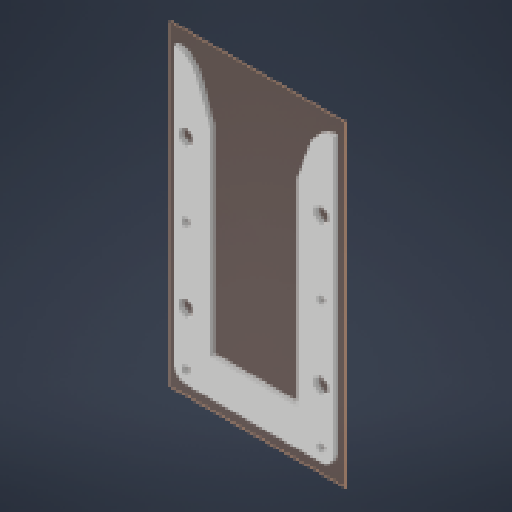
# Autodesk Inventor part: battery holder flap
Saved by Autodesk Inventor 2023 (Build 270158000, 158)
## iProperties
Created: 2022-06-04
Part Number: battery holder flap
Material: Generic
Document SubType Name: Modeling
Designer: vibhu
Density: 1 g/cm^3
Appearance: Default
Author: vibhu
Autodesk Inventor part; units mm, degrees
ref_plane "YZ Plane" through (0, 0, 0) normal (1, 0, 0) x (0, 1, 0)
ref_plane "XZ Plane" through (0, 0, 0) normal (0, 1, 0) x (-1, 0, 0)
ref_plane "XY Plane" through (0, 0, 0) normal (0, 0, 1) x (1, 0, 0)
ref_plane "Work Plane1" through (0, 0, 0) normal (0, 0, 1) x (1, 0, 0)
sketch "Sketch1" plane through (0, 0, 0) normal (0, 0, 1) x (1, 0, 0)
  line L0 (30.3146, 30.125) -> (30.3146, 26.875) projected
  line L1 (30.3146, 26.875) -> (27.5, 25.25) projected
  line L2 (27.5, 25.25) -> (24.6854, 26.875) projected
  line L3 (24.6854, 26.875) -> (24.6854, 30.125) projected
  line L4 (24.6854, 30.125) -> (27.5, 31.75) projected
  line L5 (27.5, 31.75) -> (30.3146, 30.125) projected
  line L6 (30.3146, -33.125) -> (27.5, -34.75) projected
  line L7 (27.5, -34.75) -> (24.6854, -33.125) projected
  line L8 (24.6854, -33.125) -> (24.6854, -29.875) projected
  line L9 (24.6854, -29.875) -> (27.5, -28.25) projected
  line L10 (27.5, -28.25) -> (30.3146, -29.875) projected
  line L11 (30.3146, -29.875) -> (30.3146, -33.125) projected
  line L12 (-24.6854, 26.875) -> (-27.5, 25.25) projected
  line L13 (-27.5, 25.25) -> (-30.3146, 26.875) projected
  line L14 (-30.3146, 26.875) -> (-30.3146, 30.125) projected
  line L15 (-30.3146, 30.125) -> (-27.5, 31.75) projected
  line L16 (-27.5, 31.75) -> (-24.6854, 30.125) projected
  line L17 (-24.6854, 30.125) -> (-24.6854, 26.875) projected
  line L18 (-24.6854, -33.125) -> (-27.5, -34.75) projected
  line L19 (-27.5, -34.75) -> (-30.3146, -33.125) projected
  line L20 (-30.3146, -33.125) -> (-30.3146, -29.875) projected
  line L21 (-30.3146, -29.875) -> (-27.5, -28.25) projected
  line L22 (-27.5, -28.25) -> (-24.6854, -29.875) projected
  line L23 (-24.6854, -29.875) -> (-24.6854, -33.125) projected
  line L24 (-32.5, -53.5) -> (-32.5, 58.5) projected
  arc A0 (-32.5, -53.5) -> (-27.5, -58.5) centre (-27.5, -53.5) ccw projected
  line L25 (27.5, -58.5) -> (-27.5, -58.5) projected
  arc A1 (27.5, -58.5) -> (32.5, -53.5) centre (27.5, -53.5) ccw projected
  line L26 (32.5, 58.5) -> (32.5, -53.5) projected
  arc A2 (32.5, 58.5) -> (22.5, 48.5) centre (32.5, 48.5) ccw projected
  line L27 (22.5, -48.5) -> (22.5, 48.5) projected
  line L28 (-22.5, -48.5) -> (22.5, -48.5) projected
  line L29 (-22.5, 48.5) -> (-22.5, -48.5) projected
  arc A3 (-22.5, 48.5) -> (-32.5, 58.5) centre (-32.5, 48.5) ccw projected
  circle A4 centre (27.5, -1.5) radius 1.75 projected
  circle A5 centre (-27.5, -1.5) radius 1.75 projected
  circle A6 centre (-27.5, -53.5) radius 1.75 projected
  circle A7 centre (27.5, -53.5) radius 1.75 projected
  line L30 (-17.5, -43.5) -> (17.5, -43.5)
  line L31 (17.5, -43.5) -> (17.5, 36.5259)
  line L32 (17.5, 36.5259) -> (23.1031, 51.9202)
  line L33 (-17.5, -43.5) -> (-17.5, 36.5259)
  line L34 (-17.5, 36.5259) -> (-23.1031, 51.9202)
  point P0 (0, 0)
  dimension "d0" = 5
  dimension "d1" = 5
  dimension "d2" = 5
  dimension "d3" = 20
  constraints: 10 end point, 2 point on circle, 2 tangent, 1 horizontal, 1 horizontal alignment, 1 perpendicular, 1 vertical
  measures "d0" distance between parallel lines of L28 L30
  measures "d1" distance from line of L29 L30.start
  measures "d2" distance from line of L27 L30.end
  measures "d3" angle of L34 L29
extrude "Extrusion1" add sketch "Sketch1" along normal blind 2
body "Solid1"
